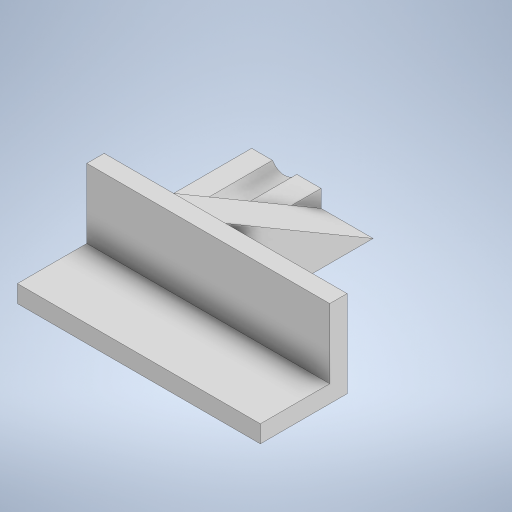
# Autodesk Inventor part: GiroMotorKrepl
Saved by Autodesk Inventor 2024 (Build 280153000, 153)
## iProperties
Created: 2023-10-17
Part Number: GiroMotorKrepl
Material: Generic
Document SubType Name: Modeling
Designer: Kippi
Density: 1 g/cm^3
Appearance: Default
Author: Kippi
Autodesk Inventor part; units mm, degrees
ref_plane "YZ Plane" through (0, 0, 0) normal (1, 0, 0) x (0, 1, 0)
ref_plane "XZ Plane" through (0, 0, 0) normal (0, 1, 0) x (-1, 0, 0)
ref_plane "XY Plane" through (0, 0, 0) normal (0, 0, 1) x (1, 0, 0)
sketch "Sketch1" plane through (0, 0, 0) normal (0, 1, 0) x (-1, 0, 0)
  line L0 (70, 85) -> (0, 85)
  line L1 (0, 85) -> (0, 0)
  line L2 (0, 0) -> (70, 0)
  line L3 (70, 0) -> (70, 85)
  line L4 (0, 0) -> (30, 0)
  line L5 (30, 0) -> (30, 80)
  line L6 (30, 80) -> (0, 80)
  line L7 (0, 80) -> (0, 0)
  dimension "d0" = 85
  dimension "d1" = 70
  dimension "d2" = 30
  dimension "d3" = 80
  constraints: 16 end point, 4 parallel, 2 horizontal, 2 perpendicular
  measures "d0" distance of L2.end L0.start
  measures "d1" distance of L0.start L0.end
  measures "d2" distance of L5.end L6.end
  measures "d3" distance of L4.end L5.end
extrude "Extrusion1" add sketch "Sketch1" along normal blind 10 contours L3 L2 L5 L6 L1 L0
sketch "Sketch2" plane through (0, 0, 85) normal (1, 0, 0) x (0, 0, -1)
  line L0 (0, 0) -> (5, 0) construction
  line L1 (0, 10) -> (5, 10) construction
  line L2 (0, 0) -> (0, 10) construction
  line L3 (-50, 0) -> (0, 0)
  line L4 (0, 0) -> (0, 50)
  line L5 (0, 50) -> (-10, 50)
  line L6 (-10, 50) -> (-10, 10)
  line L7 (-10, 10) -> (-50, 10)
  line L8 (-50, 10) -> (-50, 0)
  point P0 (85, 0)
  dimension "d6" = 50
  dimension "d7" = 50
  dimension "d8" = 40
  dimension "d9" = 40
  constraints: 12 end point, 6 perpendicular, 1 point on line
  measures "d6" distance of L0.start L4.end
  measures "d7" distance of L3.start L0.start
  measures "d8" distance of L6.end L7.end
  measures "d9" distance of L5.end L6.end
extrude "Extrusion2" add sketch "Sketch2" along normal mid plane 140
sketch "Sketch4" plane through (-30, 0, 0) normal (0, 0, -1) x (-1, 0, 0)
  circle A0 centre (21, 14) radius 8.0623
  point P0 (-30, 0)
  constraints: 1 centre point
extrude "Extrusion3" cut sketch "Sketch4" against normal blind 50
sketch "Sketch6" plane through (-30, 0, 80) normal (1, 0, 0) x (0, 0, -1)
  line L0 (-5, 50) -> (-5, 10) construction
  line L1 (80, 0) -> (-5, 50)
  line L2 (-5, 50) -> (-5, 0)
  line L3 (-5, 0) -> (80, 0)
  constraints: 6 end point, 1 collinear, 1 perpendicular
extrude "Extrusion4" add sketch "Sketch6" along normal blind 30
body "Solid1"
